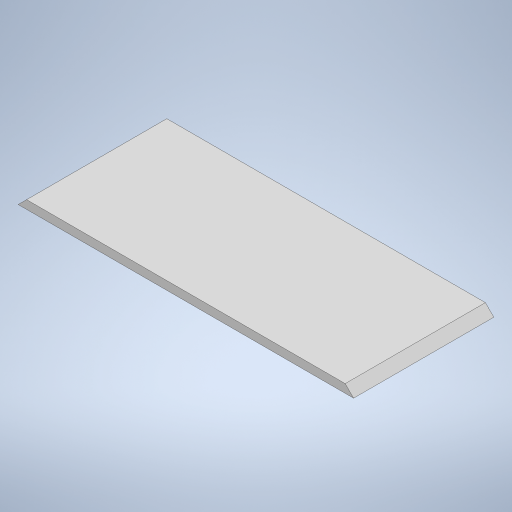
# Autodesk Inventor part: Left Wall
Saved by Autodesk Inventor 2023 (Build 270158000, 158)
## iProperties
Created: 2023-02-05
Part Number: Left Wall
Material: Generic
Document SubType Name: Modeling
Designer: Ahmed Nazir
Density: 1 g/cm^3
Appearance: Default
Author: Ahmed Nazir
Autodesk Inventor part; units mm, degrees
ref_plane "YZ Plane" through (0, 0, 0) normal (1, 0, 0) x (0, 1, 0)
ref_plane "XZ Plane" through (0, 0, 0) normal (0, 1, 0) x (-1, 0, 0)
ref_plane "XY Plane" through (0, 0, 0) normal (0, 0, 1) x (1, 0, 0)
sketch "Sketch1" plane through (0, 0, 0) normal (0, 1, 0) x (-1, 0, 0)
  line L0 (59.8, 25) -> (-59.8, 25)
  line L1 (-59.8, 25) -> (-59.8, -25)
  line L2 (-59.8, -25) -> (59.8, -25)
  line L3 (59.8, -25) -> (59.8, 25)
  line L4 (59.8, 25) -> (-59.8, -25) construction
  line L5 (-59.8, 25) -> (59.8, -25) construction
  point P0 (0, 0)
  dimension "d0" = 119.6
  dimension "d1" = 50
  constraints: 12 end point, 2 midpoint, 2 parallel, 1 horizontal, 1 perpendicular
  measures "d0" distance of L2.end L1.end
  measures "d1" distance of L1.end L0.end
extrude "Extrusion1" add sketch "Sketch1" along normal blind 3
chamfer "Chamfer1" distance 3 angle 45 1 edges at (59.8, 3, 0) measured on face at (59.8, 1, 8.3333)
chamfer "Chamfer2" distance 3 angle 45 1 edges at (-59.8, 3, 0) measured on face at (-59.8, 2, -8.3333)
body "Solid1"
